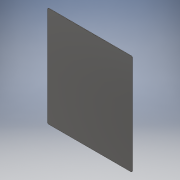
# Autodesk Inventor part: LiftBase
Saved by Autodesk Inventor 2018 (Build 220112000, 112)
## iProperties
Created: 2017-11-21
Part Number: LiftBase
Material: Steel, Galvanized
Document SubType Name: Modeling
Designer: P136265
Density: 7.85 g/cm^3
Appearance: Galvanized
Author: P136265
Autodesk Inventor part; units mm, degrees
ref_plane "YZ Plane" through (0, 0, 0) normal (1, 0, 0) x (0, 1, 0)
ref_plane "XZ Plane" through (0, 0, 0) normal (0, 1, 0) x (-1, 0, 0)
ref_plane "XY Plane" through (0, 0, 0) normal (0, 0, 1) x (1, 0, 0)
sketch "Sketch2" plane through (0, 0, 0) normal (0, 1, 0) x (-1, 0, 0)
  line L0 (-207.5, 252.5) -> (207.5, 252.5)
  line L1 (212.5, 247.5) -> (212.5, -247.5)
  line L2 (207.5, -252.5) -> (-207.5, -252.5)
  line L3 (-212.5, -247.5) -> (-212.5, 247.5)
  line L4 (-212.5, 252.5) -> (212.5, -252.5) construction
  line L5 (212.5, 252.5) -> (-212.5, -252.5) construction
  arc A0 (212.5, 247.5) -> (207.5, 252.5) centre (207.5, 247.5) ccw
  arc A1 (207.5, -252.5) -> (212.5, -247.5) centre (207.5, -247.5) ccw
  arc A2 (-207.5, 252.5) -> (-212.5, 247.5) centre (-207.5, 247.5) ccw
  arc A3 (-212.5, -247.5) -> (-207.5, -252.5) centre (-207.5, -247.5) ccw
  point P0 (0, 0)
  dimension "d10" = 425
  dimension "d11" = 505
  dimension "d12" = 5
  constraints: 12 end point, 8 point on circle, 8 point on line, 8 tangent, 4 centre point, 3 equal radius, 2 midpoint, 2 parallel, 1 horizontal, 1 perpendicular
  measures "d10" distance of L4.end L5.end
  measures "d11" distance of L5.start L4.end
  measures "d12" radius of A0
extrude "Extrusion3" add sketch "Sketch2" along normal mid plane 2
body "Solid4"
